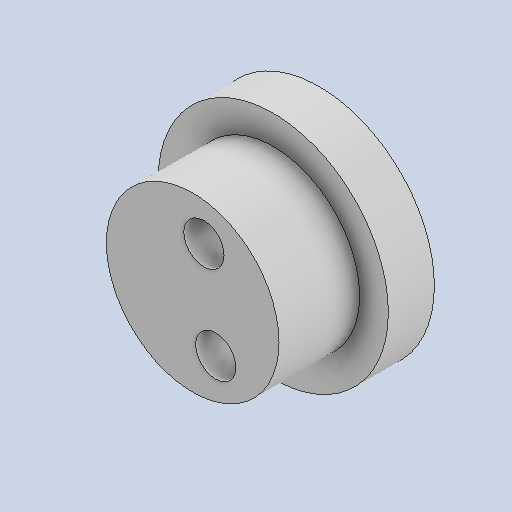
# Autodesk Inventor part: Shaft-3
Saved by Autodesk Inventor 2023 (Build 270158000, 158)
## iProperties
Created: 2023-01-17
Part Number: Shaft-3
Material: Generic
Document SubType Name: Modeling
Designer: caden
Density: 1 g/cm^3
Appearance: Default
Description: 3D Print
Author: caden
Autodesk Inventor part; units mm, degrees
ref_plane "YZ Plane" through (0, 0, 0) normal (1, 0, 0) x (0, 1, 0)
ref_plane "XZ Plane" through (0, 0, 0) normal (0, 1, 0) x (-1, 0, 0)
ref_plane "XY Plane" through (0, 0, 0) normal (0, 0, 1) x (1, 0, 0)
sketch "Sketch1" plane through (0, 0, 0) normal (0, 0, 1) x (1, 0, 0)
  circle A0 centre (19.5006, -15.159) radius 1.75 construction
  circle A1 centre (19.5006, -15.159) radius 1.75 construction
  circle A2 centre (19.5006, -15.159) radius 1.75
  circle A3 centre (20.5303, -23.0925) radius 1.75
  line L0 (19.5006, -15.159) -> (20.5303, -23.0925) construction
  line L1 (20.5303, -23.0925) -> (20.0154, -19.1258) construction
  line L2 (20.0154, -19.1258) -> (20.2426, -19.0963) construction
  circle A4 centre (18.5279, -19.3188) radius 10
  circle A5 centre (21.9301, -11.6314) radius 7.5 projected
  circle A6 centre (26.0946, -10.6293) radius 1.75 projected
  point P0 (0, 0)
  dimension "d1" = 20
  dimension "d7" = 1.5
  dimension "d8" = 8
  constraints: 6 end point, 3 centre point, 2 equal radius, 2 midpoint, 1 coincident, 1 perpendicular, 1 point on line
  measures "d1" diameter of A4
  measures "d7" distance from line of A4.centre L0
  measures "d8" distance of L0.start L0.end
extrude "Extrusion1" add sketch "Sketch1" along normal blind 4 contours A4 A5 | A5 A4 A6 | A6 A4 picked at (24.3482, -15.6706) picked at (25.0435, -11.8364)
sketch "Sketch2" plane through (18.5279, -19.3188, 4) normal (0, 0, 1) x (1, 0, 0)
  circle A0 centre (0, 0) radius 10 construction
  circle A1 centre (0, 0) radius 7.5
  circle A2 centre (0.9727, 4.1598) radius 1.75 projected
  circle A3 centre (0.9727, 4.1598) radius 1.75
  circle A4 centre (2.0024, -3.7737) radius 1.75 projected
  circle A5 centre (2.0024, -3.7737) radius 1.75
  point P0 (-18.5279, 19.3188)
  dimension "d4" = 15
  constraints: 3 centre point, 3 coincident
  measures "d4" diameter of A1
extrude "Extrusion2" add sketch "Sketch2" along normal blind 7
body "Solid1"
